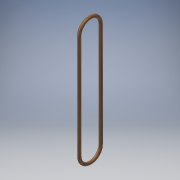
# Autodesk Inventor part: 15102898-16-P-0308
Saved by Autodesk Inventor 2017 (Build 210142000, 142)
## iProperties
Created: 2016-10-08
Part Number: 15102898-16-P-0308
Material: Polyurethane Foam
Document SubType Name: Modeling
Designer: gus
Density: 0.032 g/cm^3
Appearance: Coarse Textured - Umber
Author: gus
Autodesk Inventor part; units mm, degrees
ref_plane "YZ Plane" through (0, 0, 0) normal (1, 0, 0) x (0, 1, 0)
ref_plane "XZ Plane" through (0, 0, 0) normal (0, 1, 0) x (-1, 0, 0)
ref_plane "XY Plane" through (0, 0, 0) normal (0, 0, 1) x (1, 0, 0)
sketch "Sketch1" plane through (0, 0, 0) normal (0, 1, 0) x (-1, 0, 0)
  circle A0 centre (0, 0) radius 3.175
  dimension "d0" = 6.35
  constraints: 1 centre point, 1 coincident
  measures "d0" diameter of A0
sketch "Sketch2" plane through (0, 0, 0) normal (1, 0, 0) x (0, 1, 0)
  line L0 (0, -22.098) -> (-215.9149, -22.098) construction
  line L1 (0, 0) -> (-215.9149, 0)
  line L2 (-215.9149, -44.196) -> (0, -44.196)
  arc A0 (0, -44.196) -> (0, 0) centre (0, -22.098) ccw
  arc A1 (-215.9149, 0) -> (-215.9149, -44.196) centre (-215.9149, -22.098) ccw
  point P0 (-107.9575, -22.098)
  dimension "d1" = 215.9149
  dimension "d2" = 44.196
  constraints: 8 end point, 4 point on circle, 4 tangent, 2 centre point, 1 coincident, 1 horizontal, 1 midpoint, 1 parallel
  measures "d1" distance of L0.start L0.end
  measures "d2" diameter of A1
sweep "Sweep1" add profiles "Sketch1" path "Sketch2" path curves L1 A1 L2 A0
body "Solid1"
